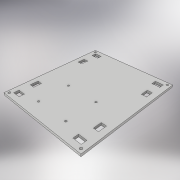
# Autodesk Inventor part: boxBottom
Saved by Autodesk Inventor 2017 (Build 210142000, 142)
## iProperties
Created: 2017-05-22
Part Number: boxBottom
Material: Generic
Document SubType Name: Modeling
Designer: Dominic Gaiero
Density: 1 g/cm^3
Appearance: Default
Author: Dominic Gaiero
Autodesk Inventor part; units mm, degrees
ref_plane "YZ Plane" through (0, 0, 0) normal (1, 0, 0) x (0, 1, 0)
ref_plane "XZ Plane" through (0, 0, 0) normal (0, 1, 0) x (-1, 0, 0)
ref_plane "XY Plane" through (0, 0, 0) normal (0, 0, 1) x (1, 0, 0)
sketch "Sketch1" plane through (0, 0, 0) normal (0, 1, 0) x (-1, 0, 0)
  line L0 (209.7643, 50.5525) -> (94.7643, 50.5525)
  line L1 (94.7643, 185.5525) -> (209.7643, 185.5525)
  line L2 (94.7643, 50.5525) -> (94.7643, 185.5525)
  line L3 (152.2643, 185.5525) -> (152.2643, 50.5525) construction
  line L4 (209.7643, 185.5525) -> (209.7643, 50.5525)
  line L5 (111.8643, 172.1025) -> (101.8643, 172.1025)
  line L6 (111.8643, 178.4525) -> (111.8643, 172.1025)
  line L7 (101.8643, 178.4525) -> (111.8643, 178.4525)
  line L8 (101.8643, 172.1025) -> (101.8643, 178.4525)
  circle A0 centre (98.7643, 181.5525) radius 1.55
  line L9 (101.8643, 158.0525) -> (108.2143, 158.0525)
  line L10 (108.2143, 158.0525) -> (108.2143, 148.0525)
  line L11 (108.2143, 148.0525) -> (101.8643, 148.0525)
  line L12 (101.8643, 148.0525) -> (101.8643, 158.0525)
  circle A1 centre (131.8808, 168.9992) radius 1.255
  line L13 (128.2613, 169.1897) -> (152.2643, 169.1897) construction
  line L14 (128.2613, 149.5681) -> (128.2613, 169.1897) construction
  line L15 (175.8733, 149.5681) -> (128.2613, 149.5681) construction
  line L16 (209.7643, 118.0525) -> (94.7643, 118.0525) construction
  line L17 (192.6643, 172.1025) -> (202.6643, 172.1025)
  line L18 (196.3143, 148.0525) -> (202.6643, 148.0525)
  line L19 (196.3143, 158.0525) -> (196.3143, 148.0525)
  line L20 (202.6643, 148.0525) -> (202.6643, 158.0525)
  line L21 (192.6643, 178.4525) -> (192.6643, 172.1025)
  line L22 (202.6643, 178.4525) -> (192.6643, 178.4525)
  line L23 (202.6643, 172.1025) -> (202.6643, 178.4525)
  circle A2 centre (205.7643, 181.5525) radius 1.55
  line L24 (202.6643, 158.0525) -> (196.3143, 158.0525)
  line L25 (108.2143, 88.0525) -> (101.8643, 88.0525)
  line L26 (101.8643, 88.0525) -> (101.8643, 78.0525)
  line L27 (101.8643, 78.0525) -> (108.2143, 78.0525)
  line L28 (111.8643, 64.0025) -> (101.8643, 64.0025)
  line L29 (101.8643, 64.0025) -> (101.8643, 57.6525)
  line L30 (111.8643, 57.6525) -> (111.8643, 64.0025)
  line L31 (101.8643, 57.6525) -> (111.8643, 57.6525)
  circle A3 centre (98.7643, 54.5525) radius 1.55
  line L32 (108.2143, 78.0525) -> (108.2143, 88.0525)
  line L33 (196.3143, 78.0525) -> (196.3143, 88.0525)
  line L34 (196.3143, 88.0525) -> (202.6643, 88.0525)
  line L35 (202.6643, 88.0525) -> (202.6643, 78.0525)
  line L36 (202.6643, 78.0525) -> (196.3143, 78.0525)
  line L37 (192.6643, 64.0025) -> (202.6643, 64.0025)
  line L38 (192.6643, 57.6525) -> (192.6643, 64.0025)
  line L39 (202.6643, 57.6525) -> (192.6643, 57.6525)
  line L40 (202.6643, 64.0025) -> (202.6643, 57.6525)
  circle A4 centre (205.7643, 54.5525) radius 1.55
  line L41 (176.2673, 169.1897) -> (152.2643, 169.1897) construction
  line L42 (176.2673, 149.5681) -> (176.2673, 169.1897) construction
  circle A5 centre (172.6478, 168.9992) radius 1.255
  line L43 (176.2673, 129.9465) -> (152.2643, 129.9465) construction
  circle A6 centre (172.6478, 130.137) radius 1.255
  line L44 (176.2673, 149.5681) -> (176.2673, 129.9465) construction
  circle A7 centre (131.8808, 130.137) radius 1.255
  line L45 (128.2613, 129.9465) -> (152.2643, 129.9465) construction
  line L46 (128.2613, 149.5681) -> (128.2613, 129.9465) construction
  circle A8 centre (144.6443, 167.7925) radius 0.9 construction
  circle A9 centre (144.6443, 165.2525) radius 0.9 construction
  circle A10 centre (144.6443, 162.7125) radius 0.9 construction
  circle A11 centre (144.6443, 160.1725) radius 0.9 construction
  circle A12 centre (144.6443, 157.6325) radius 0.9 construction
  circle A13 centre (144.6443, 155.0925) radius 0.9 construction
  circle A14 centre (144.6443, 152.5525) radius 0.9 construction
  circle A15 centre (144.6443, 150.0125) radius 0.9 construction
  circle A16 centre (144.6443, 147.4725) radius 0.9 construction
  circle A17 centre (144.6443, 144.9325) radius 0.9 construction
  circle A18 centre (144.6443, 142.3925) radius 0.9 construction
  circle A19 centre (144.6443, 139.8525) radius 0.9 construction
  circle A20 centre (159.8849, 167.7925) radius 0.9 construction
  circle A21 centre (159.8849, 165.2525) radius 0.9 construction
  circle A22 centre (159.8849, 162.7125) radius 0.9 construction
  circle A23 centre (159.8849, 160.1725) radius 0.9 construction
  circle A24 centre (159.8849, 157.6325) radius 0.9 construction
  circle A25 centre (159.8849, 155.0925) radius 0.9 construction
  circle A26 centre (159.8849, 152.5525) radius 0.9 construction
  circle A27 centre (159.8849, 150.0125) radius 0.9 construction
  circle A28 centre (159.8849, 147.4725) radius 0.9 construction
  circle A29 centre (159.8849, 144.9325) radius 0.9 construction
  circle A30 centre (159.8849, 142.3925) radius 0.9 construction
  circle A31 centre (159.8849, 139.8525) radius 0.9 construction
  line L47 (148.5143, 172.1025) -> (156.0143, 172.1025) construction
  line L48 (156.0143, 172.1025) -> (156.0143, 167.1025) construction
  line L49 (156.0143, 167.1025) -> (148.5143, 167.1025) construction
  line L50 (148.5143, 167.1025) -> (148.5143, 172.1025) construction
  line L51 (143.3743, 171.6025) -> (161.1543, 171.6025) construction
  line L52 (161.1543, 171.6025) -> (161.1543, 138.5825) construction
  line L53 (161.1543, 138.5825) -> (143.3743, 138.5825) construction
  line L54 (143.3743, 138.5825) -> (143.3743, 171.6025) construction
  line L55 (144.7643, 172.1025) -> (159.7643, 172.1025) construction
  line L56 (159.7643, 172.1025) -> (159.7643, 167.1025) construction
  line L57 (159.7643, 167.1025) -> (144.7643, 167.1025) construction
  line L58 (144.7643, 167.1025) -> (144.7643, 172.1025) construction
  line L59 (111.2143, 74.0025) -> (131.8143, 74.0025)
  line L60 (131.8143, 74.0025) -> (131.8143, 94.6025)
  line L61 (131.8143, 94.6025) -> (111.2143, 94.6025)
  line L62 (111.2143, 94.6025) -> (111.2143, 74.0025)
  line L63 (172.7143, 74.0025) -> (172.7143, 94.6025)
  line L64 (172.7143, 94.6025) -> (193.3143, 94.6025)
  line L65 (193.3143, 74.0025) -> (172.7143, 74.0025)
  line L66 (193.3143, 94.6025) -> (193.3143, 74.0025)
  line L67 (131.8143, 141.5025) -> (111.2143, 141.5025)
  line L68 (131.8143, 162.1025) -> (131.8143, 141.5025)
  line L69 (111.2143, 162.1025) -> (131.8143, 162.1025)
  line L70 (111.2143, 141.5025) -> (111.2143, 162.1025)
  line L71 (172.7143, 141.5025) -> (193.3143, 141.5025)
  line L72 (172.7143, 162.1025) -> (172.7143, 141.5025)
  line L73 (193.3143, 141.5025) -> (193.3143, 162.1025)
  line L74 (193.3143, 162.1025) -> (172.7143, 162.1025)
  point P0 (0, 0)
  point P1 (152.2643, 118.0525)
  point P2 (152.2643, 149.2659)
  point P3 (152.2643, 172.1025)
  point P4 (152.2643, 171.6025)
  point P5 (106.8643, 172.1025)
  point P6 (152.2643, 172.1025)
  dimension "d4" = 115
  dimension "d5" = 135
  dimension "d6" = 6.35
  dimension "d7" = 10
  dimension "d8" = 3.1
  dimension "d9" = 10
  dimension "d10" = 6.35
  dimension "d11" = 4
  dimension "d12" = 4
  dimension "d13" = 7.1
  dimension "d14" = 2.51
  dimension "d15" = 27.5
  dimension "d16" = 20.3835
  dimension "d17" = 19.4311
  dimension "d18" = 19.6216
  dimension "d19" = 1.8
  dimension "d20" = 16.383
  dimension "d21" = 2.54
  dimension "d22" = 15.2405
  dimension "d23" = 7.5
  dimension "d24" = 5
  dimension "d25" = 17.78
  dimension "d26" = 33.02
  dimension "d27" = 1.27
  dimension "d28" = 0.5
  dimension "d29" = 3.81
  dimension "d30" = 9.906
  dimension "d31" = 36.65
  dimension "d32" = 15
  dimension "d33" = 5
  dimension "d34" = 32.9
  dimension "d35" = 20.6
  dimension "d36" = 20.6
  dimension "d37" = 3
  dimension "d38" = 10
  dimension "d39" = 40.767
  dimension "d40" = 40.4
  dimension "d41" = 7.1
  constraints: 150 end point, 47 symmetric about line, 32 centre point, 14 parallel, 9 horizontal, 9 midpoint, 7 perpendicular, 3 vertical alignment, 2 point on line, 1 coincident, 1 horizontal alignment, 1 vertical, 52 other
  measures "d4" distance of L4.end L2.start
  measures "d5" distance of L4.start L4.end
  measures "d6" distance of L11.start L11.end
  measures "d7" distance of L9.end L11.start
  measures "d8" diameter of A0
  measures "d9" distance of L5.start L5.end
  measures "d10" distance of L6.start L5.start
  measures "d11" distance from line of L1 A0.centre
  measures "d12" distance from line of L2 A0.centre
  measures "d13" distance between parallel lines of L2 L12
  measures "d14" diameter of A1
  measures "d15" distance between parallel lines of L1 L9
  measures "d16" distance from line of L3 A1.centre
  measures "d17" distance from line of L15 A1.centre
  measures "d18" distance between parallel lines of L15 L13
  measures "d19" diameter of A8
  measures "d20" distance from line of L14 A8.centre
  measures "d21" distance of A8.centre A9.centre
  measures "d22" distance of A8.centre A20.centre
  measures "d23" distance of L49.start L49.end
  measures "d24" distance of L47.end L49.start
  measures "d25" distance of L52.end L54.start
  measures "d26" distance of L52.start L52.end
  measures "d27" distance from line of L54 A8.centre
  measures "d28" distance between parallel lines of L51 L47
  measures "d29" distance from line of L51 A8.centre
  measures "d30" distance from line of L45 A19.centre
  measures "d31" distance between parallel lines of L50 L6
  measures "d32" distance of L57.start L57.end
  measures "d33" distance of L55.end L57.start
  measures "d34" distance between parallel lines of L6 L58
  measures "d35" distance of L61.end L60.end
  measures "d36" distance of L60.end L60.start
  measures "d37" distance between parallel lines of L62 L32
  measures "d38" distance between parallel lines of L28 L59
  measures "d39" distance of A5.centre A1.centre
  measures "d40" distance between parallel lines of L3 L6
  measures "d41" distance between parallel lines of L1 L7
extrude "Extrusion2" add sketch "Sketch1" along normal blind 3.175 contours L0 L2 L1 L4 | L62 L61 L60 L59 | L63 L64 L66 L65 | L67 L70 L69 L68 | L72 L74 L73 L71
body "Solid2"
